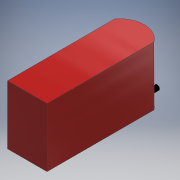
# Autodesk Inventor part: kypom_sa
Saved by Autodesk Inventor 2018 (Build 220112000, 112)
## iProperties
Created: 2018-03-07
Part Number: kypom_sa
Material: 一般
Document SubType Name: Modeling
Designer: shun
Density: 1 g/cm^3
Appearance: 既定
Author: shun
Autodesk Inventor part; units mm, degrees
ref_plane "YZ Plane" through (0, 0, 0) normal (1, 0, 0) x (0, 1, 0)
ref_plane "XZ Plane" through (0, 0, 0) normal (0, 1, 0) x (-1, 0, 0)
sketch "スケッチ1" plane through (0, 0, 0) normal (0, 0, 1) x (1, 0, 0)
  line L0 (0, 0) -> (23.5, 0)
  line L1 (23.5, 0) -> (23.5, 63.5)
  line L2 (0, 63.5) -> (0, 0)
  arc A0 (23.5, 63.5) -> (0, 63.5) centre (11.75, 54.9948) ccw
  point P0 (11.75, 69.5)
  dimension "d0" = 23.5
  dimension "d1" = 63.5
  constraints: 6 end point, 3 point on circle, 1 centre point, 1 horizontal, 1 parallel, 1 perpendicular
  measures "d0" distance of L2.start L1.end
  measures "d1" distance of L1.end L0.end
extrude "押し出し1" add sketch "スケッチ1" along normal blind 35
ref_plane "作業平面1" through (11.75, 69.5, 0) normal (0, -1, 0) x (1, 0, 0)
sketch "スケッチ2" plane through (11.75, 69.5, 0) normal (0, -1, 0) x (1, 0, 0)
  circle A0 centre (-5.4578, 1.5) radius 1.5
  circle A1 centre (2.6257, 1.5) radius 1.5
  line L0 (11.75, 0) -> (-11.75, 0) projected
  dimension "d5" = 3
  dimension "d6" = 3
  constraints: 2 centre point, 2 tangent
  measures "d5" diameter of A0
  measures "d6" diameter of A1
extrude "押し出し2" add sketch "スケッチ2" along normal mid plane 10
